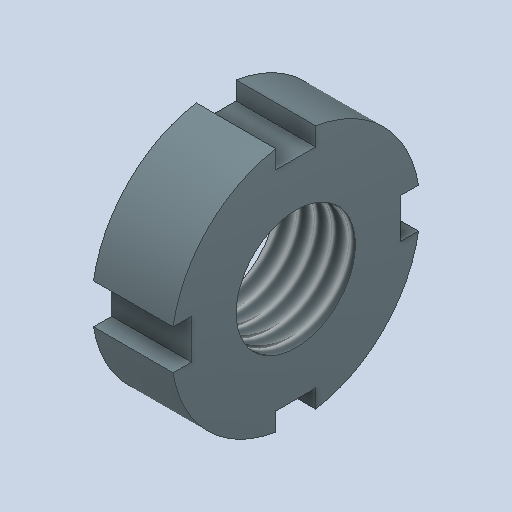
# Autodesk Inventor part: 7. LockNutM12
Saved by Autodesk Inventor 2023.2 (Build 272271030, 271C)
## iProperties
Created: 2023-03-30
Part Number: 7. LockNutM12
Material: Lead
Document SubType Name: Modeling
Designer: Luis Valente
Density: 11.34 g/cm^3
Appearance: Lead
Author: Luis Valente
Autodesk Inventor part; units mm, degrees
ref_plane "YZ Plane" through (0, 0, 0) normal (1, 0, 0) x (0, 1, 0)
ref_plane "XZ Plane" through (0, 0, 0) normal (0, 1, 0) x (-1, 0, 0)
sketch "Sketch1" plane through (0, 0, 0) normal (1, 0, 0) x (0, 1, 0)
  circle A0 centre (0, 0) radius 12.5
  dimension "d0" = 25
  constraints: 1 centre point, 1 coincident
  measures "d0" diameter of A0
extrude "Extrusion1" add sketch "Sketch1" along normal blind 8
sketch "Sketch2" plane through (8, 0, 0) normal (1, 0, 0) x (0, 0, -1)
  circle A0 centre (0, 0) radius 6
  dimension "d3" = 12
  constraints: 1 centre point, 1 coincident
  measures "d3" diameter of A0
extrude "Extrusion2" cut sketch "Sketch2" against normal blind 8
thread "Thread1" size "M12x1.75" class "6H" standard "ISO Metric profile" length 13
sketch "Sketch3" plane through (8, 0, 0) normal (1, 0, 0) x (0, 0, -1)
  circle A0 centre (0, 0) radius 12.5 projected
  line L0 (0, 12.5) -> (0, 10.5)
  line L1 (0, 10.5) -> (-2, 10.5)
  line L2 (-2, 10.5) -> (2, 10.5)
  line L3 (-2, 10.5) -> (-2, 12.339)
  line L4 (-2, 13.4004) -> (2, 13.4004)
  line L5 (2, 13.4004) -> (2, 10.5)
  line L6 (-2, 12.339) -> (-2, 13.4004)
  line L7 (-12.5, 0) -> (-10.5, 0)
  line L8 (-10.5, 0) -> (-10.5, -2)
  line L9 (-10.5, -2) -> (-10.5, 2)
  line L10 (-10.5, -2) -> (-12.339, -2)
  line L11 (-13.4004, -2) -> (-13.4004, 2)
  line L12 (-13.4004, 2) -> (-10.5, 2)
  line L13 (-12.339, -2) -> (-13.4004, -2)
  line L14 (0, -12.5) -> (0, -10.5)
  line L15 (0, -10.5) -> (2, -10.5)
  line L16 (2, -10.5) -> (-2, -10.5)
  line L17 (2, -10.5) -> (2, -12.339)
  line L18 (2, -13.4004) -> (-2, -13.4004)
  line L19 (-2, -13.4004) -> (-2, -10.5)
  line L20 (2, -12.339) -> (2, -13.4004)
  line L21 (12.5, 0) -> (10.5, 0)
  line L22 (10.5, 0) -> (10.5, 2)
  line L23 (10.5, 2) -> (10.5, -2)
  line L24 (10.5, 2) -> (12.339, 2)
  line L25 (13.4004, 2) -> (13.4004, -2)
  line L26 (13.4004, -2) -> (10.5, -2)
  line L27 (12.339, 2) -> (13.4004, 2)
  dimension "d9" = 2
  dimension "d10" = 4
  dimension "d16" = 360
  constraints: 56 end point, 8 point on line, 2 horizontal, 2 perpendicular, 2 point on circle, 2 vertical, 57 other
  measures "d9" distance of L0.end L1.end
  measures "d10" distance of L1.end L2.end
extrude "Extrusion3" cut sketch "Sketch3" against normal blind 8 contours L21 L22 L24 A0 | A0 L27 L25 L26 | A0 L26 L23 L21 | L5 L2 L0 A0 | A0 L6 L4 L5 | L20 L18 L19 A0 | A0 L14 L15 L17 | L0 L1 L3 A0 | A0 L19 L16 L14 | L12 L9 L7 A0 | A0 L13 L11 L12 | A0 L7 L8 L10
ref_plane "Work Plane1" through (0, 0, 0) normal (0, 0, 1) x (1, 0, 0)
body "Solid1"
